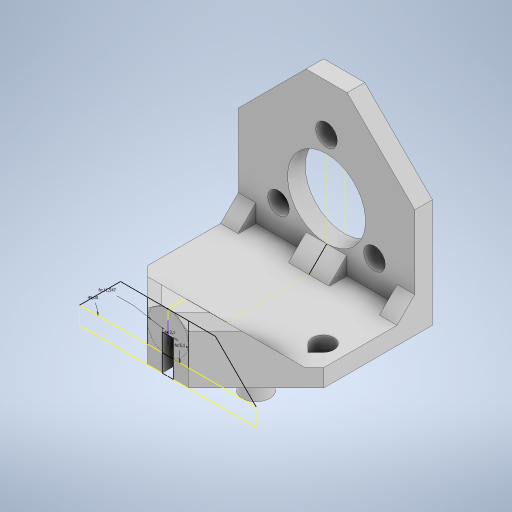
# Autodesk Inventor part: WindNacelleAltAlt
Saved by Autodesk Inventor 2024.3 (Build 283343000, 343)
## iProperties
Created: 2024-12-04
Part Number: WindNacelleAltAlt
Material: Generisch
Document SubType Name: Modeling
Designer: Maximilian Hock
Density: 1 g/cm^3
Appearance: Vorgabe
Mass: 20.6464 g
Surface Area: 106.613 cm^2
Volume: 20.6464 cm^3
Author: Maximilian Hock
## iProperties of the stored document WindNacelleAltAlt_3D-Druck.ipt
Created: 2025-02-12
Part Number: WindNacelleAltAlt_3D-Druck
Material: Generisch
Document SubType Name: Modeling
Designer: Maximilian Hock
Density: 1 g/cm^3
Appearance: Vorgabe
Author: Maximilian Hock
## iProperties of the stored document MemberDocs/x4zpnsvf4A0befcdtUtatz15uAb
Created: 2024-12-04
Part Number: WindNacelleAltAlt
Material: Generisch
Document SubType Name: Modeling
Designer: Maximilian Hock
Density: 1 g/cm^3
Appearance: Vorgabe
Mass: 20.6464 g
Surface Area: 106.613 cm^2
Volume: 20.6464 cm^3
Author: Maximilian Hock
Autodesk Inventor part; units mm, degrees
ref_plane "YZ Plane" through (0, 0, 0) normal (1, 0, 0) x (0, 1, 0)
ref_plane "XZ Plane" through (0, 0, 0) normal (0, 1, 0) x (-1, 0, 0)
ref_plane "XY Plane" through (0, 0, 0) normal (0, 0, 1) x (1, 0, 0)
sketch "Skizze1" plane through (0, 0, 0) normal (0, 0, 1) x (1, 0, 0)
  circle A0 centre (0, 0) radius 3.95
  line L0 (25, -25) -> (-25, -25)
  line L1 (-25, -25) -> (-25, 25)
  line L2 (-25, 25) -> (25, 25)
  line L3 (25, 25) -> (25, -25)
  line L4 (25, -25) -> (-25, 25) construction
  line L5 (-25, -25) -> (25, 25) construction
  circle A1 centre (19.05, 0) radius 3.05
  circle A2 centre (0, 0) radius 16 construction
  line L6 (16.8933, -2.1567) -> (19.05, -4.3134)
  line L7 (19.05, -4.3134) -> (21.2067, -2.1567)
  dimension "d2" = 7.9
  dimension "d5" = 50
  dimension "d23" = 6.1
  dimension "d24" = 32
  constraints: 16 end point, 3 centre point, 3 perpendicular, 3 tangent, 2 coincident, 2 midpoint, 2 parallel, 2 point on circle, 1 horizontal, 1 horizontal alignment, 1 vertical alignment
  measures "d2" diameter of A0
  measures "d5" distance of L0.end L1.end
  measures "d23" diameter of A1
  measures "d24" diameter of A2
extrude "Extrusion1" add sketch "Skizze1" against normal blind 16 contours A0
extrude "Extrusion2" add sketch "Skizze1" along normal blind 5 contours A0 | L0 L1 L2 L3
sketch "Skizze2" plane through (-25, 25, 0) normal (0, 1, 0) x (1, 0, 0)
  line L0 (50, 0) -> (0, 0) projected
  line L1 (0, 0) -> (0, -5) projected
  line L2 (50, -5) -> (0, -5) construction
  line L3 (50, 0) -> (50, -5) projected
  circle A0 centre (25, -36.7771) radius 5.8235 construction
  circle A1 centre (38.599, -13.2229) radius 5.8235 construction
  circle A2 centre (11.401, -13.2229) radius 5.8235 construction
  line L4 (50, -5) -> (0, -5) projected
  line L5 (0, 0) -> (50, 0) construction
  line L6 (0, -5) -> (50, -5) projected
  line L7 (0, -5) -> (0, -45)
  line L8 (0, -45) -> (50, -45)
  line L9 (50, -45) -> (50, -5)
  line L10 (19.1765, -36.7771) -> (19.1765, -50)
  line L11 (30.8235, -36.7771) -> (30.8235, -50)
  line L12 (0, 0) -> (0, -5) projected
  line L13 (0, -45) -> (50, -45) construction
  line L14 (50, -45) -> (50, -50)
  line L15 (50, -50) -> (0, -50)
  line L16 (0, -50) -> (0, -45)
  line L17 (19.1765, -50) -> (0, -30.8235)
  line L18 (30.8235, -50) -> (50, -30.8235)
  line L19 (27.9117, -31.7338) -> (30.8235, -36.7771) construction
  line L20 (30.8235, -36.7771) -> (27.9117, -41.8204) construction
  line L21 (27.9117, -41.8204) -> (22.0882, -41.8204) construction
  line L22 (22.0882, -41.8204) -> (19.1765, -36.7771) construction
  line L23 (19.1765, -36.7771) -> (22.0883, -31.7338) construction
  line L24 (22.0883, -31.7338) -> (27.9117, -31.7338) construction
  circle A3 centre (25, -21.0743) radius 11.05
  circle A4 centre (25, -36.7771) radius 3.05
  circle A5 centre (11.401, -13.2229) radius 3.05
  circle A6 centre (38.599, -13.2229) radius 3.05
  line L25 (25, -42.6006) -> (25, -45) construction
  line L26 (11.401, -7.3994) -> (11.401, -5) construction
  point P0 (25, 0)
  point P1 (25, -5)
  point P2 (0, -26.1603)
  point P3 (50, -26.1603)
  dimension "d111" = 22.1
  dimension "d8" = 11.647
  dimension "d12" = 360
  dimension "d112" = 6.1
  dimension "d115" = 50
  dimension "d116" = 50
  constraints: 38 end point, 8 point on line, 7 perpendicular, 5 centre point, 5 coincident, 4 point on circle, 3 equal length, 3 vertical, 3 vertical alignment, 2 equal radius, 2 horizontal, 2 midpoint, 2 parallel, 2 tangent, 25 other
  measures "d8" diameter of A0
  measures "d112" diameter of A4
  measures "d115" distance between parallel lines of L0 L15
  measures "d116" distance of L14.end L15.end
extrude "Extrusion3" add sketch "Skizze2" against normal blind 5 contours L9 L18 L8 L17 L7 L4 | L18 L11 L8 | L8 L10 L17 | L11 L15 L10 L8
sketch "Skizze3" plane through (-25, -25, 0) normal (0, -1, 0) x (1, 0, 0)
  line L0 (0, 0) -> (50, 0) projected
  line L1 (50, 0) -> (50, 5) projected
  line L2 (0, 5) -> (50, 5) projected
  line L3 (0, 0) -> (0, 5) projected
  line L4 (0, 5) -> (11.547, 16.547)
  line L5 (11.547, 16.547) -> (38.453, 16.547)
  line L6 (38.453, 16.547) -> (50, 5)
  circle A0 centre (25, 10.7735) radius 5.7735 construction
  line L7 (0, 5) -> (50, 5) projected
  line L8 (19.2265, 5) -> (19.2265, 16.547)
  line L9 (30.7735, 5) -> (30.7735, 16.547)
  line L10 (26.55, 5) -> (23.45, 5)
  line L11 (23.45, 5) -> (23.45, 10.1)
  line L12 (23.45, 10.1) -> (26.55, 10.1)
  line L13 (26.55, 10.1) -> (26.55, 5)
  line L14 (23.45, 5) -> (26.55, 5)
  line L15 (26.55, 5) -> (26.55, 0)
  line L16 (26.55, 0) -> (23.45, 0)
  line L17 (23.45, 0) -> (23.45, 5)
  point P0 (25, 0)
  point P1 (25, 16.547)
  point P2 (25, 5)
  point P3 (25, 5)
  point P4 (19.2265, 5)
  point P5 (25, 5)
  point P6 (26.55, 5)
  dimension "d18" = 11.547
  dimension "d20" = 45
  dimension "d132" = 3.1
  dimension "d133" = 5.1
  constraints: 26 end point, 6 point on line, 5 midpoint, 4 parallel, 4 perpendicular, 4 tangent, 3 horizontal, 2 vertical alignment, 1 centre point
  measures "d18" diameter of A0
  measures "d20" angle of L2 L4
  measures "d132" distance of L11.end L12.end
  measures "d133" distance of L12.end L10.start
extrude "Extrusion4" add sketch "Skizze3" against normal blind 5 contours L3 L2 L17 L0 | L17 L2 L15 L0 | L15 L2 L1 L0 | L2 L8 L5 L9 L13 L12 L11
sketch "Skizze9" plane through (0, 0, 5) normal (0, 0, 1) x (1, 0, 0)
  line L0 (25, -25) -> (25, 20) projected
  line L1 (25, 20) -> (-25, 20) projected
  line L2 (-25, 20) -> (-25, -25) projected
  line L3 (-25, -25) -> (-5.7735, -25) projected
  line L4 (-5.7735, -25) -> (-5.7735, -20) projected
  line L5 (-5.7735, -20) -> (-1.55, -20) projected
  line L6 (5.7735, -20) -> (5.7735, -25) projected
  line L7 (5.7735, -25) -> (25, -25) projected
  arc A0 (21.2067, -2.1567) -> (16.8933, -2.1567) centre (19.05, 0) ccw projected
  line L8 (-5.7735, -25) -> (-25, -5.7735)
  line L9 (5.7735, -25) -> (25, -5.7735)
  line L10 (21.2067, -2.1567) -> (19.05, -4.3134) projected
  line L11 (19.05, -4.3134) -> (16.8933, -2.1567) projected
  line L12 (-1.55, -20) -> (-1.55, -25) projected
  line L13 (-1.55, -25) -> (1.55, -25) projected
  line L14 (1.55, -25) -> (1.55, -20) projected
  line L15 (1.55, -20) -> (5.7735, -20) projected
  point P0 (0, 0)
  dimension "d76" = 45
  constraints: 4 end point, 2 point on line, 1 perpendicular
  measures "d76" angle of L3 L8
extrude "Extrusion12" cut sketch "Skizze9" against normal through all contours L7 L9 L0 | L8 L3 L2
chamfer "Fasen10" distance 2 angle 45 1 edges at (-3.95, 0, 0)
sketch "Skizze15" plane through (0, 0, 0) normal (1, 0, 0) x (0, 1, 0)
  line L0 (-25, 7.7235) -> (-25, 13.8235)
  line L1 (-25, 5) -> (-5.7735, 5) construction
  line L2 (-5.7735, 5) -> (20, 5) construction
  line L3 (20, 5) -> (-5.7735, 5) construction
  line L4 (-5.7735, 5) -> (-25, 5) construction
  line L5 (-25, 5) -> (-20, 5) construction
  line L6 (-20, 5) -> (-25, 5) construction
  line L7 (-2.1567, 5) -> (-4.3134, 5) construction
  line L8 (-4.3134, 5) -> (-2.1567, 5) construction
  line L9 (-2.1567, 5) -> (-2.1567, 5) construction
  line L10 (20, 10.0243) -> (20, 32.1243) construction
  line L11 (25, 32.1243) -> (25, 10.0243) construction
  line L12 (-20, 16.547) -> (-8.453, 5)
  line L13 (-20, 5) -> (-20, 16.547)
  line L14 (-20, 5) -> (-8.453, 5)
  line L15 (20, 10.0243) -> (14.9757, 5)
  line L16 (20, 5) -> (14.9757, 5)
  line L17 (20, 5) -> (20, 10.0243)
  line L18 (-20, 5) -> (-25, 5) projected
  line L19 (-25, 5) -> (-20, 5) projected
  line L20 (-25, 5) -> (-25, 16.547) projected
  line L21 (-20, 5) -> (-25, 5) projected
  line L22 (-20, 16.547) -> (-20, 5) projected
  line L23 (-25, 16.547) -> (-20, 16.547) projected
  point P0 (0, 0)
  constraints: 12 end point, 3 perpendicular, 2 point on line, 1 collinear
extrude "Extrusion17" add sketch "Skizze15" against normal blind 5 from surface at 25 contours L17 L16 L15
extrude "Extrusion18" add sketch "Skizze15" along normal up to surface (5.7735 mm away) contours L17 L16 L15
sketch "Skizze16" plane through (-5.7735, -25, 16.547) normal (0, 0, 1) x (1, 0, 0)
  line L0 (11.547, 0) -> (11.547, 5) projected
  line L1 (11.547, 5) -> (16.547, 5)
  line L2 (30.7735, 19.2265) -> (11.547, 0) projected
  line L3 (11.547, 0) -> (11.547, 5)
  line L4 (11.547, 0) -> (0, 0) projected
  line L5 (11.547, 0) -> (16.547, 5)
  line L6 (0, 0) -> (0, 5) projected
  line L7 (0, 0) -> (0, 5)
  line L8 (0, 5) -> (-5, 5)
  line L9 (-19.2265, 19.2265) -> (0, 0) projected
  line L10 (-5, 5) -> (0, 0)
  point P0 (5.7735, 25)
  constraints: 12 end point, 2 collinear, 2 perpendicular, 1 horizontal, 1 point on line
extrude "Extrusion20" add sketch "Skizze16" against normal through all
extrude "Extrusion21" add sketch "Skizze15" along normal up to surface from surface at 1.55 contours L13 L12 L14 surface through (5.7735, -25, 5) normal (-0.7071068, 0.7071068, 0)
mirror "Spiegeln4" about plane through (0, 0, 0) normal (1, 0, 0) of "Extrusion17", "Extrusion18", "Extrusion21"
chamfer "Fasen11" distance 2.724 angle 45 2 edges at (8.2735, -22.5, 16.547) (-8.2735, -22.5, 16.547)
extrude "Extrusion22" cut sketch "Skizze3" against normal blind 3 contours L17 L2 L15 L0
sketch "Skizze17" plane through (0, 0, 0) normal (0, 0, -1) x (-1, 0, 0)
  line L0 (-5.3975, 22.4369) -> (5.3975, 22.4369) construction
  line L1 (5.3975, 22.4369) -> (5.3975, 19.4654) construction
  line L2 (5.3975, 19.4654) -> (-5.3975, 19.4654) construction
  line L3 (-5.3975, 19.4654) -> (-5.3975, 22.4369) construction
  line L4 (-2.4704, 18.8688) -> (-5.0429, 18.8688)
  line L5 (-5.0429, 18.8688) -> (-5.0429, 19.4389)
  spline S0 degree 2 poles (-5.0429, 19.4389) (-4.7168, 19.6998) (-4.1949, 20.1593) (-3.9992, 20.3664) knots 0 0 0 1 2 2 2
  spline S1 degree 2 poles (-3.9992, 20.3664) (-3.7411, 20.6358) (-3.5113, 21.0471) (-3.5113, 21.2626) knots 0 0 0 1 2 2 2
  spline S2 degree 2 poles (-3.5113, 21.2626) (-3.5113, 21.5065) (-3.8035, 21.7675) (-4.0644, 21.7675) knots 0 0 0 1 2 2 2
  spline S3 degree 2 poles (-4.0644, 21.7675) (-4.1977, 21.7675) (-4.436, 21.7023) (-4.5579, 21.6512) knots 0 0 0 1 2 2 2
  spline S4 degree 2 poles (-4.5579, 21.6512) (-4.6771, 21.5973) (-4.8472, 21.4839) (-4.8898, 21.4555) knots 0 0 0 1 2 2 2
  line L6 (-4.8898, 21.4555) -> (-4.9579, 21.4555)
  line L7 (-4.9579, 21.4555) -> (-4.9579, 22.2185)
  spline S5 degree 2 poles (-4.9579, 22.2185) (-4.8104, 22.2894) (-4.1807, 22.4369) (-3.8886, 22.4369) knots 0 0 0 1 2 2 2
  spline S6 degree 2 poles (-3.8886, 22.4369) (-3.2646, 22.4369) (-2.6236, 21.8809) (-2.6236, 21.3789) knots 0 0 0 1 2 2 2
  spline S7 degree 2 poles (-2.6236, 21.3789) (-2.6236, 21.0698) (-2.9157, 20.4741) (-3.2532, 20.1338) knots 0 0 0 1 2 2 2
  spline S8 degree 2 poles (-3.2532, 20.1338) (-3.466, 19.9239) (-3.8659, 19.5977) (-3.9538, 19.5296) knots 0 0 0 1 2 2 2
  line L8 (-3.9538, 19.5296) -> (-2.4704, 19.5296)
  line L9 (-2.4704, 19.5296) -> (-2.4704, 18.8688)
  line L10 (-1.1657, 18.8688) -> (-1.9968, 18.8688)
  line L11 (-1.9968, 18.8688) -> (-1.9968, 19.7934)
  line L12 (-1.9968, 19.7934) -> (-1.1657, 19.7934)
  line L13 (-1.1657, 19.7934) -> (-1.1657, 18.8688)
  line L14 (1.9429, 18.8688) -> (-0.3687, 18.8688)
  line L15 (-0.3687, 18.8688) -> (-0.3687, 19.4786)
  line L16 (-0.3687, 19.4786) -> (0.3687, 19.4786)
  line L17 (0.3687, 19.4786) -> (0.3687, 21.3307)
  line L18 (0.3687, 21.3307) -> (-0.3687, 21.3307)
  line L19 (-0.3687, 21.3307) -> (-0.3687, 21.9008)
  spline S9 degree 2 poles (-0.3687, 21.9008) (-0.2071, 21.9008) (0.1135, 21.9433) (0.2099, 21.9887) knots 0 0 0 1 2 2 2
  spline S10 degree 2 poles (0.2099, 21.9887) (0.3205, 22.0454) (0.4453, 22.2355) (0.4566, 22.3773) knots 0 0 0 1 2 2 2
  line L20 (0.4566, 22.3773) -> (1.2224, 22.3773)
  line L21 (1.2224, 22.3773) -> (1.2224, 19.4786)
  line L22 (1.2224, 19.4786) -> (1.9429, 19.4786)
  line L23 (1.9429, 19.4786) -> (1.9429, 18.8688)
  line L24 (3.4036, 18.8688) -> (2.5725, 18.8688)
  line L25 (2.5725, 18.8688) -> (2.5725, 19.7934)
  line L26 (2.5725, 19.7934) -> (3.4036, 19.7934)
  line L27 (3.4036, 19.7934) -> (3.4036, 18.8688)
  line L28 (6.5122, 18.8688) -> (4.2006, 18.8688)
  line L29 (4.2006, 18.8688) -> (4.2006, 19.4786)
  line L30 (4.2006, 19.4786) -> (4.938, 19.4786)
  line L31 (4.938, 19.4786) -> (4.938, 21.3307)
  line L32 (4.938, 21.3307) -> (4.2006, 21.3307)
  line L33 (4.2006, 21.3307) -> (4.2006, 21.9008)
  spline S11 degree 2 poles (4.2006, 21.9008) (4.3622, 21.9008) (4.6827, 21.9433) (4.7792, 21.9887) knots 0 0 0 1 2 2 2
  spline S12 degree 2 poles (4.7792, 21.9887) (4.8898, 22.0454) (5.0146, 22.2355) (5.0259, 22.3773) knots 0 0 0 1 2 2 2
  line L34 (5.0259, 22.3773) -> (5.7917, 22.3773)
  line L35 (5.7917, 22.3773) -> (5.7917, 19.4786)
  line L36 (5.7917, 19.4786) -> (6.5122, 19.4786)
  line L37 (6.5122, 19.4786) -> (6.5122, 18.8688)
  point P0 (0, 0)
  point P1 (0, 19.4654)
  constraints: 1 midpoint, 1 vertical alignment, 2 other
emboss "Prägen1" sketch "Skizze17" operation cut depth 0.5 direction (0, 0, 1)
equation "\"d24\" = WindTowerOuterDiameter"
equation "\"d18\" = HexnutOuterSize"
equation "\"WindTowerOuterDiameter\" = 32"
equation "\"HexnutOuterSize\" = 11.547"
